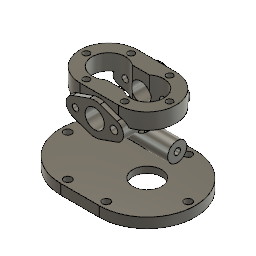
Task2e v0 (Autodesk Fusion 360 design; units mm, degrees)
Autodesk Fusion 360 part; units mm, degrees
note: some values were not read from the file. Set by a fixed rule: which sketch regions a step uses.
sketch "Sketch1" plane through (0, 0, 0) normal (0, 1, 0) x (1, 0, 0)
  line L0 (-30, 75) -> (30, 75)
  arc A0 (30, -75) -> (30, 75) centre (30, 0) ccw
  arc A1 (-30, 75) -> (-30, -75) centre (-30, 0) ccw
  line L1 (30, -75) -> (-30, -75)
  constraint horizontal L0
  constraint tangent L0 A0
  constraint tangent A1 L1
extrude "Extrude1" add sketch "Sketch1" along normal blind 16 makes body 1
sketch "Sketch2" plane through (0, 16, 0) normal (0, 1, 0) x (-1, 0, 0)
  arc A0 (30, -75) -> (30, 75) centre (30, 0) ccw
  line L0 (30, 75) -> (-30, 75)
  arc A1 (-30, 75) -> (-30, -75) centre (-30, 0) ccw
  line L1 (-30, -75) -> (30, -75)
  circle A2 centre (30, -64) radius 6
  circle A3 centre (-30, -64) radius 6
  circle A4 centre (-94, 0) radius 6
  circle A5 centre (94, 0) radius 6
  circle A6 centre (30, 64) radius 6
  circle A7 centre (-30, 64) radius 6
extrude "Extrude2" cut sketch "Sketch2" against normal through all contours A2 | A3 | A4 | A5 | A6 | A7 bodies 1
sketch "Sketch3" plane through (0, 16, 0) normal (0, 1, 0) x (-1, 0, 0)
  circle A0 centre (-30, 64) radius 6
  circle A1 centre (30, -64) radius 6
  circle A2 centre (30, 64) radius 6
  circle A3 centre (-94, 0) radius 6
  circle A4 centre (-30, -64) radius 6
  circle A5 centre (94, 0) radius 6
  arc A6 (30, -75) -> (30, 75) centre (30, 0) ccw
  line L0 (30, 75) -> (-30, 75)
  arc A7 (-30, 75) -> (-30, -75) centre (-30, 0) ccw
  line L1 (-30, -75) -> (30, -75)
  circle A8 centre (-30, 0) radius 38
  constraint concentric A7 A8
extrude "Extrude3" cut sketch "Sketch3" against normal through all contours A8 bodies 1
sketch "Sketch10" plane through (0, 16, 0) normal (0, 1, 0) x (-1, 0, 0)
  circle A0 centre (-30, 0) radius 38
  circle A1 centre (-30, 64) radius 6
  circle A2 centre (30, -64) radius 6
  circle A3 centre (30, 64) radius 6
  circle A4 centre (-94, 0) radius 6
  circle A5 centre (-30, -64) radius 6
  circle A6 centre (94, 0) radius 6
  arc A7 (30, -75) -> (30, 75) centre (30, 0) ccw
  line L0 (30, 75) -> (-30, 75)
  arc A8 (-30, 75) -> (-30, -75) centre (-30, 0) ccw
  line L1 (-30, -75) -> (30, -75)
  circle A9 centre (-30, 0) radius 38
  constraint concentric A0 A9
extrude "Extrude8" add sketch "Sketch10" against normal blind 10 contours A0 A9 bodies 1
sketch "Sketch7" plane through (0, 0, 0) normal (0, 1, 0) x (1, 0, 0)
  line L0 (-30, 45) -> (30, 45)
  arc A0 (-30, 45) -> (-30, -45) centre (-30, 0) ccw
  arc A1 (30, -45) -> (30, 45) centre (30, 0) ccw
  line L1 (30, -45) -> (-30, -45)
  constraint tangent L0 A0
  constraint tangent A0 L1
extrude "Extrude5" add sketch "Sketch7" along normal blind 25 separate body makes body 2
sketch "Sketch8" plane through (0, 25, 0) normal (0, 1, 0) x (-1, 0, 0)
  arc A0 (30, -45) -> (30, 45) centre (30, 0) ccw
  line L0 (30, 45) -> (-30, 45)
  arc A1 (-30, 45) -> (-30, -45) centre (-30, 0) ccw
  line L1 (-30, -45) -> (30, -45)
  circle A2 centre (65, 0) radius 5
  circle A3 centre (-30, -35) radius 5
  circle A4 centre (-30, 35) radius 5
  circle A5 centre (30, 35) radius 5
  circle A6 centre (30, -35) radius 5
  circle A7 centre (-65, 0) radius 5
extrude "Extrude6" cut sketch "Sketch8" against normal blind 16 contours A2 | A3 | A4 | A5 | A6 | A7 bodies 2
sketch "Sketch9" plane through (0, 25, 0) normal (0, 1, 0) x (-1, 0, 0)
  circle A0 centre (-30, 35) radius 5
  circle A1 centre (30, -35) radius 5
  circle A2 centre (30, 35) radius 5
  circle A3 centre (-65, 0) radius 5
  circle A4 centre (-30, -35) radius 5
  circle A5 centre (65, 0) radius 5
  arc A6 (30, -45) -> (30, 45) centre (30, 0) ccw
  line L0 (30, 45) -> (-30, 45)
  arc A7 (-30, 45) -> (-30, -45) centre (-30, 0) ccw
  line L1 (-30, -45) -> (30, -45)
  line L2 (0, -20) -> (-13.3868, -20)
  line L3 (13.3868, -20) -> (0, -20)
  line L4 (0, 20) -> (13.3868, 20)
  line L5 (0, 20) -> (-13.3868, 20)
  arc A8 (13.3868, -20) -> (13.3868, 20) centre (30, 0) ccw
  arc A9 (-13.3868, 20) -> (-13.3868, -20) centre (-30, 0) ccw
  constraint parallel L4 L5
extrude "Extrude7" cut sketch "Sketch9" against normal through all contours L2 L3 L4 L5 A8 A9 bodies 2
move_body "Move1" bodies 2 to x (1, 0, 0) y (0, 1, 0) z (0, 0, 1) at (0, 112, 0)
sketch "Sketch13" plane through (0, 16, 0) normal (0, 1, 0) x (-1, 0, 0)
  circle A0 centre (-30, 64) radius 6
  circle A1 centre (30, -64) radius 6
  circle A2 centre (30, 64) radius 6
  circle A3 centre (-94, 0) radius 6
  circle A4 centre (-30, -64) radius 6
  circle A5 centre (94, 0) radius 6
  arc A6 (30, -75) -> (30, 75) centre (30, 0) ccw
  line L0 (30, 75) -> (-30, 75)
  arc A7 (-30, 75) -> (-30, -75) centre (-30, 0) ccw
  line L1 (-30, -75) -> (30, -75)
  line L2 (-30, -64) -> (-30, 64)
  circle A8 centre (-30, 0) radius 22.5
  dimension "d62" = 45
  constraint coincident A4.centre L2.start
  constraint coincident A0.centre L2.end
  constraint concentric A7 A8
  measures "d62" diameter of A8
extrude "Extrude9" cut sketch "Sketch13" against normal through all contours L2 A8 | L2 A8 bodies 1
sketch "Sketch15" plane through (0, 0, 45) normal (0, 0, 1) x (1, 0, 0)
  line L0 (-30, 112) -> (30, 112)
  line L1 (30, 112) -> (30, 137)
  line L2 (30, 137) -> (-30, 137)
  line L3 (-30, 137) -> (-30, 112)
  line L4 (0, 137) -> (0, 107) construction
  circle A0 centre (0, 107) radius 15
  circle A1 centre (-30, 107) radius 5
  circle A2 centre (30, 107) radius 6
  line L5 (-35, 121.1421) -> (-8.3333, 130.5702)
  line L6 (35, 121.1421) -> (8.3333, 130.5702)
  line L7 (-35, 92.8579) -> (-8.3333, 83.4298)
  line L8 (8.3333, 83.4298) -> (35, 92.8579)
  arc A3 (-35, 121.1421) -> (-35, 92.8579) centre (-30, 107) ccw
  arc A4 (-8.3333, 83.4298) -> (8.3333, 83.4298) centre (0, 107) ccw
  arc A5 (35, 92.8579) -> (35, 121.1421) centre (30, 107) ccw
  arc A6 (8.3333, 130.5702) -> (-8.3333, 130.5702) centre (0, 107) ccw
  constraint midpoint L2 L4.start
  constraint coincident L4.end A0.centre
extrude "Extrude10" add sketch "Sketch15" along normal blind 7 contours L0 L1 L3 A0 A2 L5 L6 A6 | L0 L1 L3 A0 A2 L5 L6 L7 L8 A3 A4 A5 bodies 2
mirror "Mirror1" about plane through (0, 0, 0) normal (0, 0, 1) of "Extrude10"
extrude "Extrude11" cut 1 faces at (2.3587, 118.6878, 45) along direction (0, 0, -1) through all on bodies 2 bodies 2
extrude "Extrude12" cut 1 faces at (29.7082, 112.6453, 45) along direction (0, 0, -1) through all on bodies 2 bodies 2
extrude "Extrude13" add 1 faces at (-18.3462, 91.3025, 45) along direction (0, 0, -1) blind 95 on bodies 2 bodies 2
sketch "Sketch16" plane through (0, 137, 0) normal (0, 1, 0) x (-1, 0, 0)
  arc A0 (13.3868, -20) -> (13.3868, 20) centre (30, 0) ccw
  line L0 (13.3868, -20) -> (-13.3868, -20)
  arc A1 (-13.3868, 20) -> (-13.3868, -20) centre (-30, 0) ccw
  line L1 (-13.3868, 20) -> (13.3868, 20)
  circle A2 centre (-30, 35) radius 5
  circle A3 centre (30, -35) radius 5
  circle A4 centre (30, 35) radius 5
  circle A5 centre (-65, 0) radius 5
  circle A6 centre (-30, -35) radius 5
  circle A7 centre (65, 0) radius 5
  arc A8 (30, -45) -> (30, 45) centre (30, 0) ccw
  line L2 (30, 45) -> (-30, 45)
  arc A9 (-30, 45) -> (-30, -45) centre (-30, 0) ccw
  line L3 (-30, -45) -> (30, -45)
extrude "Extrude14" cut sketch "Sketch16" against normal blind 60 contours A0 L0 A1 L1 bodies 2
sketch "Sketch17" plane through (0, 0, 0) normal (1, 0, 0) x (0, 0, -1)
  line L0 (0, 0) -> (0, 4.0573)
  circle A0 centre (0, 75.0573) radius 15
  circle A1 centre (0, 75.0573) radius 5
  dimension "d81" = 30
  dimension "d82" = 10
  constraint coincident L0.start origin
  constraint vertical L0
  constraint concentric A0 A1
  measures "d81" diameter of A0
  measures "d82" diameter of A1
extrude "Extrude15" add sketch "Sketch17" along normal mid plane 154 separate body makes body 3
sketch "Sketch18" plane through (0, 137, 0) normal (0, 1, 0) x (-1, 0, 0)
  arc A0 (13.3868, -20) -> (13.3868, 20) centre (30, 0) ccw
  line L0 (13.3868, -20) -> (-13.3868, -20)
  arc A1 (-13.3868, 20) -> (-13.3868, -20) centre (-30, 0) ccw
  line L1 (-13.3868, 20) -> (13.3868, 20)
  circle A2 centre (-30, 35) radius 5
  circle A3 centre (30, -35) radius 5
  circle A4 centre (30, 35) radius 5
  circle A5 centre (-65, 0) radius 5
  circle A6 centre (-30, -35) radius 5
  circle A7 centre (65, 0) radius 5
  arc A8 (30, -45) -> (30, 45) centre (30, 0) ccw
  line L2 (30, 45) -> (-30, 45)
  arc A9 (-30, 45) -> (-30, -45) centre (-30, 0) ccw
  line L3 (-30, -45) -> (30, -45)
  circle A10 centre (-30, 0) radius 12.5
  circle A11 centre (30, 0) radius 12.5
  line L4 (30, -12.5) -> (-30, -12.5)
  line L5 (30, 12.5) -> (-30, 12.5)
  dimension "d85" = 25
  dimension "d86" = 25
  constraint concentric A1 A10
  constraint concentric A0 A11
  constraint coincident A11 L4.start
  constraint coincident A10 L4.end
  constraint tangent A10 L4
  constraint horizontal L4
  constraint coincident A11 L5.start
  constraint coincident A10 L5.end
  constraint tangent A10 L5
  constraint parallel L4 L5
  measures "d85" diameter of A10
  measures "d86" diameter of A11
extrude "Extrude16" cut sketch "Sketch18" against normal blind 100 contours A10 | A10 A11 L4 L5 | A11 bodies 3
sketch "Sketch14" plane through (0, 0, 0) normal (0, 0, 1) x (1, 0, 0)
sketch "Sketch12" plane through (0, 0, 0) normal (0, 0, 1) x (1, 0, 0)
sketch "Sketch11" plane through (0, 16, 0) normal (0, 1, 0) x (-1, 0, 0)
  circle A0 centre (-30, 64) radius 6
  circle A1 centre (30, -64) radius 6
  circle A2 centre (30, 64) radius 6
  circle A3 centre (-94, 0) radius 6
  circle A4 centre (-30, -64) radius 6
  circle A5 centre (94, 0) radius 6
  arc A6 (30, -75) -> (30, 75) centre (30, 0) ccw
  line L0 (30, 75) -> (-30, 75)
  arc A7 (-30, 75) -> (-30, -75) centre (-30, 0) ccw
  line L1 (-30, -75) -> (30, -75)
  line L2 (-30, -64) -> (-30, 64)
  line L3 (36, -64) -> (36, 64)
  circle A8 centre (-30, 0) radius 38
  line L4 (30, -64) -> (30, 64)
  circle A9 centre (30, 0) radius 25
  dimension "d57" = 76
  dimension "d58" = 50
  constraint coincident A4.centre L2.start
  constraint coincident A0.centre L2.end
  constraint coincident A1 L3.start
  constraint coincident A2 L3.end
  constraint tangent A2 L3
  constraint vertical L3
  constraint concentric A7 A8
  constraint coincident A1.centre L4.start
  constraint coincident A2.centre L4.end
  constraint concentric A6 A9
  measures "d57" diameter of A8
  measures "d58" diameter of A9
